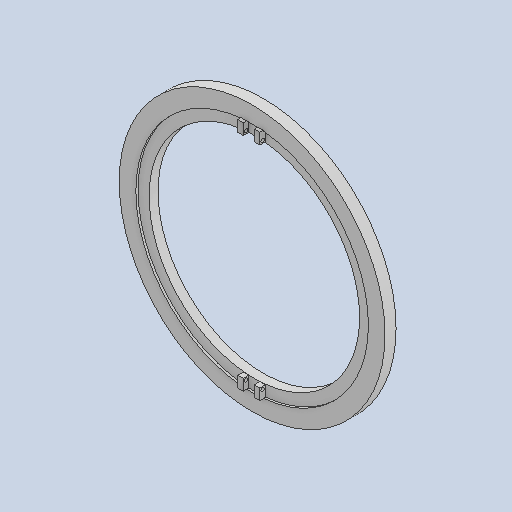
# Autodesk Inventor part: Top opening
Saved by Autodesk Inventor 2025.2 (Build 292293000, 293)
## iProperties
Created: 2025-06-02
Part Number: Top opening
Material: Generic
Document SubType Name: Modeling
Designer: dylan
Density: 1 g/cm^3
Appearance: Default
Author: dylan
Autodesk Inventor part; units mm, degrees
ref_plane "YZ Plane" through (0, 0, 0) normal (1, 0, 0) x (0, 1, 0)
ref_plane "XZ Plane" through (0, 0, 0) normal (0, 1, 0) x (-1, 0, 0)
ref_plane "XY Plane" through (0, 0, 0) normal (0, 0, 1) x (1, 0, 0)
sketch "Sketch1" plane through (0, 0, 0) normal (0, 0, 1) x (1, 0, 0)
  circle A0 centre (0, 0) radius 600
  circle A1 centre (0, 0) radius 575
  circle A2 centre (0, 0) radius 525
  circle A3 centre (0, 0) radius 475
  dimension "d2" = 1200
  dimension "d1" = 1150
  dimension "d0" = 1050
  dimension "d9" = 950
  constraints: 4 centre point, 4 coincident
  measures "d2" diameter of A0
  measures "d1" diameter of A1
  measures "d0" diameter of A2
  measures "d9" diameter of A3
extrude "Extrusion1" add sketch "Sketch1" along normal blind 50 contours A0 | A1 | A2 | A3
extrude "Extrusion2" cut sketch "Sketch1" along normal blind 20 contours A1
extrude "Extrusion3" cut sketch "Sketch1" along normal blind 315.5 contours A3
sketch "Sketch3" plane through (0, 0, 0) normal (0, 0, 1) x (1, 0, 0)
  circle A0 centre (0, 0) radius 475 projected
  line L0 (475, 0) -> (525, 0)
  circle A1 centre (0, 0) radius 525 projected
  line L1 (500, 0) -> (500, 50)
  line L2 (500, 50) -> (430, 50)
  line L3 (430, 50) -> (430, -50)
  line L4 (430, -50) -> (500, -50)
  line L5 (500, -50) -> (500, 50)
  line L6 (0, -117.9134) -> (0, 153.6807)
  line L7 (-500, 50) -> (-430, 50)
  line L8 (-430, 50) -> (-430, -50)
  line L9 (-430, -50) -> (-500, -50)
  line L10 (-500, -50) -> (-500, 50)
  line L11 (465, 0) -> (465, 25)
  line L12 (465, 25) -> (-465, 25)
  line L13 (-465, 25) -> (-465, -25)
  line L14 (-465, -25) -> (465, -25)
  line L15 (465, -25) -> (465, 25)
  point P0 (472.3611, -50)
  point P1 (472.3611, 50)
  point P2 (430, -25)
  point P3 (430, 25)
  point P4 (-430, -25)
  point P5 (-430, 25)
  dimension "d12" = 50
  dimension "d13" = 70
  dimension "d14" = 100
  dimension "d17" = 50
  constraints: 32 end point, 4 parallel, 4 symmetric about line, 3 horizontal, 3 vertical, 2 perpendicular, 1 horizontal alignment, 1 midpoint, 3 other
  measures "d12" distance of L1.start L1.end
  measures "d13" distance of L4.end L3.end
  measures "d14" distance of L3.end L2.end
  measures "d17" distance of L13.end L12.end
extrude "Extrusion4" [suppressed]
sketch "Sketch4" plane through (-472.3611, 50, 0) normal (0, 1, 0) x (1, 0, 0)
  line L0 (42.3611, 0) -> (42.3611, -50) projected
  line L1 (42.3611, -50) -> (24.8611, -50) construction
  line L2 (42.3611, -50) -> (0, -50) projected
  line L3 (24.8611, -50) -> (24.8611, -25) construction
  line L4 (42.3611, 0) -> (0, 0) projected
  line L5 (24.8611, -50) -> (49.8611, -50) construction
  circle A0 centre (24.8611, -25) radius 7.9375
  point P0 (472.3611, 0)
  dimension "d18" = 17.5
  dimension "d19" = 25
  dimension "d20" = 90
  dimension "d21" = 15.875
  constraints: 6 end point, 2 perpendicular, 1 centre point, 1 coincident, 1 horizontal, 1 point on line
  measures "d18" distance of L0.end L1.end
  measures "d19" distance of L1.end L3.end
  measures "d20" angle of L5 L3
  measures "d21" diameter of A0
extrude "Extrusion5" [suppressed]
sketch "Sketch5" plane through (430, 50, 0) normal (0, 1, 0) x (1, 0, 0)
  line L0 (42.3611, -50) -> (0, -50) projected
  line L1 (0, -50) -> (0, -25) construction
  line L2 (0, 0) -> (0, -50) projected
  line L3 (42.3611, 0) -> (42.3611, -50) projected
  line L4 (0, -25) -> (21.1805, -25) construction
  circle A0 centre (21.1805, -25) radius 7.9375
  point P0 (-430, 0)
  dimension "d25" = 21.1806
  dimension "d26" = 15.875
  constraints: 4 end point, 1 centre point, 1 coincident, 1 midpoint
  measures "d25" distance of L1.end L4.end
  measures "d26" diameter of A0
extrude "Extrusion6" [suppressed]
sketch "Sketch6" plane through (0, 0, 50) normal (0, 0, 1) x (1, 0, 0)
  circle A0 centre (0, 0) radius 525
  constraints: 1 centre point, 1 coincident
extrude "Extrusion7" cut sketch "Sketch6" against normal blind 10
sketch "Sketch7" plane through (0, 0, 40) normal (0, 0, 1) x (1, 0, 0)
  circle A0 centre (0, 0) radius 475 projected
  circle A1 centre (0, 0) radius 600 projected
  line L0 (0, 475) -> (-290.4738, 475)
  line L1 (-290.4738, 475) -> (-290.4738, 525)
  line L2 (-290.4738, 525) -> (0, 525)
  line L3 (0, 525) -> (0, 475)
  line L4 (0, 475) -> (291, 475)
  line L5 (291, 475) -> (291, 525)
  line L6 (291, 525) -> (0, 525)
  line L7 (0, 525) -> (0, 475)
  line L8 (0, 475) -> (25, 475)
  line L9 (25, 475) -> (0, 475)
  line L10 (0, 475) -> (-25, 475)
  line L11 (-50, 475) -> (-25, 475)
  line L12 (-25, 475) -> (-25, 525)
  line L13 (-25, 525) -> (-50, 525)
  line L14 (-50, 525) -> (-50, 475)
  line L15 (25, 475) -> (50, 475)
  line L16 (50, 475) -> (50, 525)
  line L17 (50, 525) -> (25, 525)
  line L18 (25, 525) -> (25, 475)
  dimension "d31" = 50
  dimension "d32" = 50
  dimension "d33" = 25
  dimension "d34" = 25
  dimension "d35" = 25
  dimension "d36" = 25
  dimension "d37" = 50
  dimension "d38" = 25
  dimension "d39" = 50
  constraints: 38 end point, 8 parallel, 5 horizontal, 4 perpendicular, 3 point on line, 1 collinear, 1 vertical alignment, 3 other
  measures "d31" distance of L0.end L1.end
  measures "d32" distance of L5.end L4.end
  measures "d33" distance of L0.start L8.end
  measures "d34" distance of L8.end L0.start
  measures "d35" distance of L0.start L10.end
  measures "d36" distance of L10.end L11.start
  measures "d37" distance of L13.end L11.start
  measures "d38" distance of L17.end L16.end
  measures "d39" distance of L16.end L15.end
extrude "Extrusion8" add sketch "Sketch7" along normal blind 25 contours L0 L14 L2 L12 | L18 L6 L16 L4
sketch "Sketch8" plane through (-25, 475, 40) normal (1, 0, 0) x (0, 0, -1)
  line L0 (-25, 0) -> (-12.5, 0) construction
  line L1 (-12.5, 0) -> (-12.5, 12.5) construction
  circle A0 centre (-12.5, 12.5) radius 7.9375
  point P0 (40, -475)
  dimension "d42" = 12.5
  dimension "d43" = 12.5
  dimension "d44" = 15.875
  constraints: 4 end point, 1 centre point, 1 coincident, 1 horizontal, 1 perpendicular, 1 point on line
  measures "d42" distance of L0.start L0.end
  measures "d43" distance of L0.end L1.end
  measures "d44" diameter of A0
extrude "Extrusion9" cut sketch "Sketch8" along normal blind 75 and the other way blind 25
mirror "Mirror1" about plane through (0, 0, 0) normal (0, 1, 0) of "Extrusion8"
sketch "Sketch9" plane through (-50, -525, 65) normal (-1, 0, 0) x (0, 0, 1)
  line L0 (-25, 50) -> (0, 50) projected
  line L1 (0, 50) -> (-12.5, 50) construction
  line L2 (-12.5, 50) -> (-12.5, 37.5) construction
  line L3 (-25, 50) -> (-25, 0.5956) projected
  line L4 (-12.5, 50) -> (0, 50) construction
  circle A0 centre (-12.5, 37.5) radius 7.9375
  point P0 (-65, 525)
  dimension "d49" = 12.5
  dimension "d50" = 90
  dimension "d51" = 15.875
  constraints: 6 end point, 1 centre point, 1 coincident, 1 horizontal, 1 midpoint, 1 parallel, 1 perpendicular
  measures "d49" distance of L1.end L2.end
  measures "d50" angle of L2 L4
  measures "d51" diameter of A0
extrude "Extrusion10" cut sketch "Sketch9" against normal up to surface (100 mm away)
body "Solid1"
